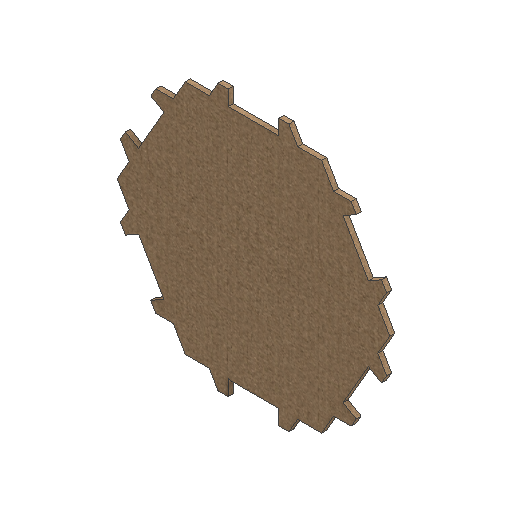
# Autodesk Inventor part: middle_space_3
Saved by Autodesk Inventor 2024 (Build 280153000, 153)
## iProperties
Created: 2024-03-28
Part Number: middle_space_3
Material: MDF Medium Density Fiberboard
Document SubType Name: Modeling
Designer: op04o
Density: 0.8 g/cm^3
Appearance: Cardboard - Corrugated
Mass: 42.9665 g
Surface Area: 377.714 cm^2
Volume: 53.7081 cm^3
Author: op04o
Autodesk Inventor part; units mm, degrees
ref_plane "YZ Plane" through (0, 0, 0) normal (1, 0, 0) x (0, 1, 0)
ref_plane "XZ Plane" through (0, 0, 0) normal (0, 1, 0) x (-1, 0, 0)
ref_plane "XY Plane" through (0, 0, 0) normal (0, 0, 1) x (1, 0, 0)
sketch "Sketch1" plane through (0, 0, 0) normal (0, 0, 1) x (1, 0, 0)
  line L0 (-15, 73) -> (15, 73)
  line L1 (15, 73) -> (15, 70)
  line L2 (-15, 70) -> (-15, 73)
  line L3 (-40.4145, 70) -> (-15, 70)
  line L4 (15, 70) -> (40.4145, 70)
  line L5 (-70.7199, 23.5096) -> (-55.7199, 49.4904)
  line L6 (-55.7199, 49.4904) -> (-53.1218, 47.9904)
  line L7 (-68.1218, 22.0096) -> (-70.7199, 23.5096)
  line L8 (-55.7199, -49.4904) -> (-70.7199, -23.5096)
  line L9 (-70.7199, -23.5096) -> (-68.1218, -22.0096)
  line L10 (-53.1218, -47.9904) -> (-55.7199, -49.4904)
  line L11 (15, -73) -> (-15, -73)
  line L12 (-15, -73) -> (-15, -70)
  line L13 (15, -70) -> (15, -73)
  line L14 (70.7199, -23.5096) -> (55.7199, -49.4904)
  line L15 (55.7199, -49.4904) -> (53.1218, -47.9904)
  line L16 (68.1218, -22.0096) -> (70.7199, -23.5096)
  line L17 (55.7199, 49.4904) -> (70.7199, 23.5096)
  line L18 (70.7199, 23.5096) -> (68.1218, 22.0096)
  line L19 (53.1218, 47.9904) -> (55.7199, 49.4904)
  line L20 (-80.829, 0) -> (-68.1218, 22.0096)
  line L21 (-53.1218, 47.9904) -> (-40.4145, 70)
  line L22 (40.4145, 70) -> (53.1218, 47.9904)
  line L23 (68.1218, 22.0096) -> (80.829, 0)
  line L24 (80.829, 0) -> (68.1218, -22.0096)
  line L25 (53.1218, -47.9904) -> (40.4145, -70)
  line L26 (40.4145, -70) -> (15, -70)
  line L27 (-15, -70) -> (-40.4145, -70)
  line L28 (-40.4145, -70) -> (-53.1218, -47.9904)
  line L29 (-68.1218, -22.0096) -> (-80.829, 0)
  line L30 (15, 70) -> (-15, 70)
  line L31 (-53.1218, 47.9904) -> (-68.1218, 22.0096)
  line L32 (-68.1218, -22.0096) -> (-53.1218, -47.9904)
  line L33 (-15, -70) -> (15, -70)
  line L34 (53.1218, -47.9904) -> (68.1218, -22.0096)
  line L35 (68.1218, 22.0096) -> (53.1218, 47.9904)
  line L36 (-15, 73) -> (-15, 79)
  line L37 (-15, 79) -> (-21, 79)
  line L38 (-21, 79) -> (-21, 70)
  line L39 (15, 73) -> (15, 79)
  line L40 (15, 79) -> (21, 79)
  line L41 (21, 79) -> (21, 70)
  line L42 (-55.7199, 49.4904) -> (-60.916, 52.4904)
  line L43 (-57.916, 57.6865) -> (-50.1218, 53.1865)
  line L44 (-60.916, 52.4904) -> (-57.916, 57.6865)
  line L45 (-70.7199, 23.5096) -> (-75.916, 26.5096)
  line L46 (-75.916, 26.5096) -> (-78.916, 21.3135)
  line L47 (-78.916, 21.3135) -> (-71.1218, 16.8135)
  line L48 (-70.7199, -23.5096) -> (-75.916, -26.5096)
  line L49 (-78.916, -21.3135) -> (-71.1218, -16.8135)
  line L50 (-75.916, -26.5096) -> (-78.916, -21.3135)
  line L51 (-55.7199, -49.4904) -> (-60.916, -52.4904)
  line L52 (-60.916, -52.4904) -> (-57.916, -57.6865)
  line L53 (-57.916, -57.6865) -> (-50.1218, -53.1865)
  line L54 (-15, -73) -> (-15, -79)
  line L55 (-21, -79) -> (-21, -70)
  line L56 (-15, -79) -> (-21, -79)
  line L57 (15, -73) -> (15, -79)
  line L58 (15, -79) -> (21, -79)
  line L59 (21, -79) -> (21, -70)
  line L60 (55.7199, -49.4904) -> (60.916, -52.4904)
  line L61 (57.916, -57.6865) -> (50.1218, -53.1865)
  line L62 (60.916, -52.4904) -> (57.916, -57.6865)
  line L63 (70.7199, -23.5096) -> (75.916, -26.5096)
  line L64 (75.916, -26.5096) -> (78.916, -21.3135)
  line L65 (78.916, -21.3135) -> (71.1218, -16.8135)
  line L66 (70.7199, 23.5096) -> (75.916, 26.5096)
  line L67 (78.916, 21.3135) -> (71.1218, 16.8135)
  line L68 (75.916, 26.5096) -> (78.916, 21.3135)
  line L69 (55.7199, 49.4904) -> (60.916, 52.4904)
  line L70 (60.916, 52.4904) -> (57.916, 57.6865)
  line L71 (57.916, 57.6865) -> (50.1218, 53.1865)
  line L72 (-21, 79) -> (-26.1962, 70)
  line L73 (21, 79) -> (26.1962, 70)
  line L74 (-57.916, 57.6865) -> (-47.5237, 57.6865)
  line L75 (-78.916, 21.3135) -> (-73.7199, 12.3135)
  line L76 (-78.916, -21.3135) -> (-73.7199, -12.3135)
  line L77 (-57.916, -57.6865) -> (-47.5237, -57.6865)
  line L78 (-21, -79) -> (-26.1962, -70)
  line L79 (21, -79) -> (26.1962, -70)
  line L80 (57.916, -57.6865) -> (47.5237, -57.6865)
  line L81 (78.916, -21.3135) -> (73.7199, -12.3135)
  line L82 (78.916, 21.3135) -> (73.7199, 12.3135)
  line L83 (57.916, 57.6865) -> (47.5237, 57.6865)
  point P0 (0, 0)
  point P1 (0, 0)
  point P2 (0, 73)
  point P3 (-63.2199, 36.5)
  point P4 (-63.2199, -36.5)
  point P5 (0, -73)
  point P6 (63.2199, -36.5)
  point P7 (63.2199, 36.5)
  point P8 (71.1218, 16.8135)
  point P9 (50.1218, -53.1865)
  point P10 (71.1218, -16.8135)
  point P11 (21, -70)
  point P12 (-71.1218, -16.8135)
  point P13 (-50.1218, -53.1865)
  point P14 (-71.1218, 16.8135)
  point P15 (-50.1218, 53.1865)
  point P16 (-47.5237, 57.6865)
  point P17 (-73.7199, 12.3135)
  point P18 (-73.7199, -12.3135)
  point P19 (-47.5237, -57.6865)
  point P20 (-26.1962, -70)
  point P21 (26.1962, -70)
  point P22 (47.5237, -57.6865)
  point P23 (73.7199, -12.3135)
  point P24 (73.7199, 12.3135)
  point P25 (47.5237, 57.6865)
  dimension "d1" = 3
  dimension "d3" = 30
  dimension "d6" = 360
  dimension "d8" = 140
  dimension "d9" = 146
  dimension "d14" = 360
  dimension "d16" = 6
  dimension "d17" = 6
  dimension "d18" = 6
  dimension "d19" = 6
  dimension "d22" = 360
  dimension "d24" = 60
  dimension "d25" = 60
  dimension "d28" = 360
  constraints: 168 end point, 16 point on line, 4 perpendicular, 3 horizontal, 1 coincident, 1 midpoint, 1 parallel, 1 vertical, 1 vertical alignment, 197 other
  measures "d1" distance of L2.start L0.start
  measures "d3" distance of L0.start L0.end
  measures "d8" distance between parallel lines of L27 L3
  measures "d9" distance between parallel lines of L14 L5
  measures "d16" distance of L0.start L36.end
  measures "d17" distance of L36.end L37.end
  measures "d18" distance of L0.end L39.end
  measures "d19" distance of L39.end L40.end
  measures "d24" angle of L3 L72
  measures "d25" angle of L4 L73
extrude "Extrusion1" add sketch "Sketch1" along normal blind 3 contours L2 L3 L38 L37 L36 | L39 L40 L41 L4 L1 | L30 L4 L22 L35 L23 L24 L34 L25 L26 L33 L27 L28 L32 L29 L20 L31 L21 L3 | L3 L72 L38 | L41 L73 L4 | L21 L43 L74 | L83 L71 L22 | L21 L6 L42 L44 L43 | L71 L70 L69 L19 L22 | L20 L47 L46 L45 L7 | L18 L66 L68 L67 L23 | L20 L75 L47 | L67 L82 L23 | L29 L49 L76 | L81 L65 L24 | L29 L9 L48 L50 L49 | L65 L64 L63 L16 L24 | L28 L53 L52 L51 L10 | L15 L60 L62 L61 L25 | L28 L77 L53 | L61 L80 L25 | L27 L55 L78 | L79 L59 L26 | L27 L12 L54 L56 L55 | L59 L58 L57 L13 L26
body "Solid1"
